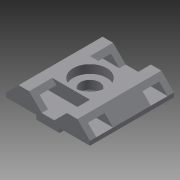
# Autodesk Inventor part: harness clip
Saved by Autodesk Inventor 2015 SP1 (Build 190203100, 203)
## iProperties
Created: 2015-02-19
Part Number: harness clip
Material: Generic
Document SubType Name: Modeling
Designer: Joseph
Density: 1 g/cm^3
Appearance: Default
Author: Joseph
Autodesk Inventor part; units mm, degrees
ref_plane "YZ Plane" through (0, 0, 0) normal (1, 0, 0) x (0, 1, 0)
ref_plane "XZ Plane" through (0, 0, 0) normal (0, 1, 0) x (-1, 0, 0)
ref_plane "XY Plane" through (0, 0, 0) normal (0, 0, 1) x (1, 0, 0)
sketch "Sketch1" plane through (0, 0, 0) normal (0, 0, 1) x (1, 0, 0)
  line L0 (10, 10) -> (-10, 10)
  line L1 (-10, 10) -> (-10, -10)
  line L2 (-10, -10) -> (10, -10)
  line L3 (10, -10) -> (10, 10)
  line L4 (10, 10) -> (-10, -10) construction
  line L5 (-10, 10) -> (10, -10) construction
  dimension "d0" = 20
  dimension "d1" = 20
  constraints: 12 end point, 2 parallel, 1 horizontal, 1 perpendicular
  measures "d0" distance of L2.end L1.end
  measures "d1" distance of L1.end L0.end
extrude "Extrusion1" add sketch "Sketch1" along normal blind 4
chamfer "Chamfer7" distance 3 angle 45 2 edges at (10, 0, 4) (-10, 0, 4)
sketch "Sketch2" plane through (0, 0, 0) normal (0, 0, -1) x (-1, 0, 0)
  line L0 (2, 1.1547) -> (2, -1.1547) projected
  line L1 (2, -1.1547) -> (0, -2.3094) projected
  line L2 (0, -2.3094) -> (-2, -1.1547) projected
  line L3 (-2, -1.1547) -> (-2, 1.1547) projected
  line L4 (-2, 1.1547) -> (0, 2.3094) projected
  line L5 (0, 2.3094) -> (2, 1.1547) projected
  line L6 (10, -10) -> (-10, -10) projected
  line L7 (-2.75, 10) -> (2.75, 10)
  line L8 (2.75, 10) -> (2.75, -10)
  line L9 (2.75, -10) -> (-2.75, -10)
  line L10 (-2.75, -10) -> (-2.75, 10)
  line L11 (-2.75, 10) -> (2.75, -10) construction
  line L12 (2.75, 10) -> (-2.75, -10) construction
  point P0 (0, 0)
  dimension "d5" = 5.5
  constraints: 12 end point, 2 midpoint, 2 parallel, 1 horizontal, 1 perpendicular, 1 point on line
  measures "d5" distance of L8.end L9.end
extrude "Extrusion2" add sketch "Sketch2" along normal blind 1
sketch "Sketch3" plane through (0, 0, -1) normal (0, 0, -1) x (-1, 0, 0)
  line L0 (2, -1.1547) -> (0, -2.3094) projected
  line L1 (0, -2.3094) -> (-2, -1.1547) projected
  line L2 (-2, -1.1547) -> (-2, 1.1547) projected
  line L3 (-2, 1.1547) -> (0, 2.3094) projected
  line L4 (0, 2.3094) -> (2, 1.1547) projected
  line L5 (2, 1.1547) -> (2, -1.1547) projected
  line L6 (-2.75, 2.75) -> (2.75, 2.75)
  line L7 (2.75, 2.75) -> (2.75, -2.75)
  line L8 (2.75, -2.75) -> (-2.75, -2.75)
  line L9 (-2.75, -2.75) -> (-2.75, 2.75)
  line L10 (-2.75, 2.75) -> (2.75, -2.75) construction
  line L11 (2.75, 2.75) -> (-2.75, -2.75) construction
  point P0 (0, 0)
  dimension "d8" = 5.5
  dimension "d9" = 5.5
  constraints: 12 end point, 2 midpoint, 2 parallel, 1 horizontal, 1 perpendicular
  measures "d8" distance of L7.end L8.end
  measures "d9" distance of L6.end L7.end
extrude "Extrusion3" cut sketch "Sketch3" against normal up to surface (1 mm away) from surface at 0
sketch "Sketch8" plane through (0, 0, 4) normal (0, 0, 1) x (1, 0, 0)
  line L0 (-7, -10) -> (7, -10) projected
  line L1 (7, 10) -> (-7, 10) projected
  line L2 (-1.5, -10) -> (1.5, -10)
  line L3 (1.5, -10) -> (1.5, -4.5)
  line L4 (1.5, -4.5) -> (-1.5, -4.5)
  line L5 (-1.5, -4.5) -> (-1.5, -10)
  line L6 (-1.5, 10) -> (1.5, 10)
  line L7 (1.5, 10) -> (1.5, 4.5)
  line L8 (1.5, 4.5) -> (-1.5, 4.5)
  line L9 (-1.5, 4.5) -> (-1.5, 10)
  line L10 (-1.5, -10) -> (-1.5, 10) construction
  line L11 (1.5, -10) -> (1.5, 10) construction
  line L12 (-1.5, 4.5) -> (0, 0) construction
  line L13 (0, 0) -> (1.5, -4.5) construction
  dimension "d82" = 9
  dimension "d83" = 3
  constraints: 24 end point, 10 point on line, 4 parallel, 4 perpendicular, 2 collinear, 2 horizontal
  measures "d82" distance between parallel lines of L4 L8
  measures "d83" distance between parallel lines of L11 L10
extrude "Extrusion7" cut sketch "Sketch8" against normal blind 3
chamfer "Chamfer8" distance 3 angle 45 4 edges at (-1.5, 7.25, 4) (-1.5, -7.25, 4) (1.5, -7.25, 4) (1.5, 7.25, 4)
sketch "Sketch9" plane through (10, -10, 0) normal (1, 0, 0) x (0, 0, -1)
  line L0 (-4, 5.5) -> (-1, 5.5) projected
  line L1 (-1, 14.5) -> (-4, 14.5) projected
  line L2 (-1, 5.5) -> (-3, 5.5)
  line L3 (-3, 5.5) -> (-3, 1.5)
  line L4 (-3, 1.5) -> (-1, 1.5)
  line L5 (-1, 1.5) -> (-1, 5.5)
  line L6 (-1, 14.5) -> (-3, 14.5)
  line L7 (-3, 14.5) -> (-3, 18.5)
  line L8 (-3, 18.5) -> (-1, 18.5)
  line L9 (-1, 18.5) -> (-1, 14.5)
  point P0 (0, 10)
  dimension "d69" = 2
  dimension "d70" = 4
  dimension "d71" = 2
  dimension "d72" = 4
  constraints: 16 end point, 4 parallel, 2 horizontal, 2 perpendicular
  measures "d69" distance of L4.end L3.end
  measures "d70" distance of L3.end L2.end
  measures "d71" distance of L7.end L8.end
  measures "d72" distance of L6.end L7.end
extrude "Extrusion8" cut sketch "Sketch9" against normal through all
sketch "Sketch10" plane through (0, 0, 4) normal (0, 0, 1) x (1, 0, 0)
  point P0 (0, 0)
  point P1 (0, 0)
  constraints: 1 coincident
hole "Hole2" at (0, 0, 4) direction (0, 0, -1) diameter 4.5 end through all counterbore diameter 8 counterbore depth 2 clearance for "Socket Head Cap Screw" size "M4" standard "Ansi Metric M Profile"
body "Solid1"
